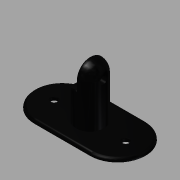
# Autodesk Inventor part: anclaje panel 2 parte panel
Saved by Autodesk Inventor 2014 (Build 180170000, 170)
## iProperties
Created: 2016-11-10
Part Number: anclaje panel 2 parte panel
Material: UHMW, Black
Document SubType Name: Modeling
Designer: Cristian
Density: 0.94 g/cm^3
Appearance: Smooth - Black
Author: Cristian
Autodesk Inventor part; units mm, degrees
ref_plane "YZ Plane" through (0, 0, 0) normal (1, 0, 0) x (0, 1, 0)
ref_plane "XZ Plane" through (0, 0, 0) normal (0, 1, 0) x (-1, 0, 0)
ref_plane "XY Plane" through (0, 0, 0) normal (0, 0, 1) x (1, 0, 0)
sketch "Sketch1" plane through (0, 0, 0) normal (0, 0, 1) x (1, 0, 0)
  line L0 (-25, -30) -> (25, -30) construction
  line L1 (25, -30) -> (25, 30) construction
  line L2 (25, 30) -> (-25, 30) construction
  line L3 (-25, 30) -> (-25, -30) construction
  line L4 (-25, -30) -> (25, 30) construction
  line L5 (25, -30) -> (-25, 30) construction
  line L6 (-25, 30) -> (-17.3178, 20.7813) construction
  line L7 (25, 30) -> (17.3178, 20.7813) construction
  line L8 (0, 0) -> (25.8269, 0) construction
  circle A0 centre (-17.3178, 20.7813) radius 2.5 construction
  circle A1 centre (17.3178, 20.7813) radius 2.5 construction
  circle A2 centre (-17.3178, -20.7813) radius 2.5 construction
  circle A3 centre (17.3178, -20.7813) radius 2.5 construction
  line L9 (-40, -20) -> (40, -20)
  line L10 (40, -20) -> (40, 20)
  line L11 (40, 20) -> (-40, 20)
  line L12 (-40, 20) -> (-40, -20)
  line L13 (-40, -20) -> (40, 20) construction
  line L14 (40, -20) -> (-40, 20) construction
  line L15 (0, 0) -> (30, 0) construction
  circle A4 centre (25.8269, 0) radius 2.35
  line L16 (0, 0) -> (0, -16.6985) construction
  line L17 (0, 0) -> (-30, 0) construction
  circle A5 centre (-25.8269, 0) radius 2.35
  dimension "d0" = 50
  dimension "d1" = 60
  dimension "d2" = 12
  dimension "d3" = 12
  dimension "d4" = 5
  dimension "d5" = 5
  dimension "d37" = 80
  dimension "d38" = 40
  dimension "d39" = 30
  dimension "d40" = 4.7
  constraints: 36 end point, 6 centre point, 4 midpoint, 4 parallel, 4 symmetric about line, 3 coincident, 3 horizontal, 3 point on line, 2 perpendicular, 1 vertical, 3 other
  measures "d0" distance of L2.end L1.end
  measures "d1" distance of L1.end L0.end
  measures "d2" distance of L2.end L6.end
  measures "d3" distance of L1.end L7.end
  measures "d4" diameter of A0
  measures "d5" diameter of A1
  measures "d37" distance of L11.end L10.end
  measures "d38" distance of L10.end L9.end
  measures "d39" distance of L8.start L15.end
  measures "d40" diameter of A4
sketch "Sketch6" plane through (0, 0, 0) normal (1, 0, 0) x (0, 1, 0)
  line L0 (-30, 2) -> (30, 2) projected
  line L1 (0, 2) -> (0, 12) construction
  line L2 (-10, 32) -> (-10, -8) construction
  line L3 (-10, -8) -> (10, -8) construction
  line L4 (10, -8) -> (10, 32) construction
  line L5 (10, 32) -> (-10, 32) construction
  line L6 (-10, 32) -> (10, -8) construction
  line L7 (-10, -8) -> (10, 32) construction
  line L8 (0, 32) -> (0, 12) construction
  circle A0 centre (0, 22) radius 10 construction
  line L9 (-10, 22) -> (-10, -8)
  line L10 (-10, -8) -> (10, -8)
  line L11 (10, -8) -> (10, 22)
  arc A1 (10, 22) -> (-10, 22) centre (0, 22) ccw
  circle A2 centre (0, 22) radius 2.5
  point P0 (0, 0)
  dimension "d20" = 10
  dimension "d21" = 20
  dimension "d22" = 5
  constraints: 22 end point, 6 point on circle, 5 midpoint, 4 vertical, 3 centre point, 3 tangent, 2 parallel, 2 point on line, 1 coincident, 1 horizontal, 1 perpendicular
  measures "d20" distance of L1.start L1.end
  measures "d21" distance of L3.end L2.end
  measures "d22" diameter of A2
extrude "Extrusion6" add sketch "Sketch6" along normal mid plane 20
fillet "Fillet1" radius 9.5 6 edges at (10, 0, 32) (10, 10, 7) (10, -10, 7) (-10, 0, 32) (-10, 10, 7) (-10, -10, 7)
sketch "Sketch8" plane through (0, 0, 0) normal (1, 0, 0) x (0, 1, 0)
  arc A0 (2.5, 22) -> (-2.5, 22) centre (0, 22) ccw projected
  circle A1 centre (0, 22) radius 11
  point P0 (0, 0)
  dimension "d27" = 22
  constraints: 1 centre point, 1 coincident
  measures "d27" diameter of A1
extrude "Extrusion7" cut sketch "Sketch8" against normal blind 20
fillet "Fillet2" radius 1 3 edges at (0, -10, 19.7087) (0, 10, 19.7087) (0, 0, 32)
fillet "Fillet3" radius 1 7 edges at (-10, 0, 11) (-6.6287, 7.7587, 14.2024) (0, 10, 17.4174) (0.78, 9.9959, 17.4084) (0, -10, 17.4174) (0.78, -9.9959, 17.4084) (-6.6294, -7.7581, 14.2018)
sketch "Sketch10" plane through (0.5, 10, -8) normal (0, 0, -1) x (-1, 0, 0)
  line L0 (-39.5, 10) -> (40.5, 10) projected
  line L1 (-39.5, -30) -> (-39.5, 10) projected
  line L2 (40.5, -30) -> (-39.5, -30) projected
  line L3 (40.5, 10) -> (40.5, -30) projected
  circle A0 centre (26.3269, -10) radius 2.35 projected
  circle A1 centre (-25.3269, -10) radius 2.35 projected
  point P0 (0.5, -10)
extrude "Extrusion9" add sketch "Sketch10" along normal blind 2.3
fillet "Fillet7" radius 0.5 2 edges at (-23.4769, 0, -8) (28.1769, 0, -8)
fillet "Fillet8" radius 20 4 edges at (40, -20, -9.15) (40, 20, -9.15) (-40, 20, -9.15) (-40, -20, -9.15)
fillet "Fillet9" radius 2 8 edges at (-34.1422, 14.1422, -8) (-40, 0, -8) (-34.1422, -14.1422, -8) (0, -20, -8) (34.1422, 14.1422, -8) (40, 0, -8) (34.1422, -14.1422, -8) (0, 20, -8)
body "Solid1"
